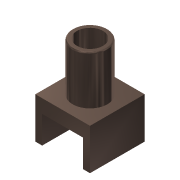
# Autodesk Inventor part: suporte-barra
Saved by Autodesk Inventor 2015 (Build 190159000, 159)
## iProperties
Created: 2016-08-11
Part Number: suporte-barra
Material: Steel, Carbon
Document SubType Name: Modeling
Designer: EriveltonDell
Density: 7.87 g/cm^3
Appearance: Gunmetal - Antique Polished
Mass: 377.778 g
Surface Area: 137.801 cm^2
Volume: 48.0022 cm^3
Author: EriveltonDell
Autodesk Inventor part; units mm, degrees
ref_plane "YZ Plane" through (0, 0, 0) normal (1, 0, 0) x (0, 1, 0)
ref_plane "XZ Plane" through (0, 0, 0) normal (0, 1, 0) x (-1, 0, 0)
ref_plane "XY Plane" through (0, 0, 0) normal (0, 0, 1) x (1, 0, 0)
sketch "Sketch1" plane through (0, 0, 0) normal (0, 1, 0) x (-1, 0, 0)
  line L0 (15, 0) -> (20, 0)
  line L1 (20, 0) -> (20, 20)
  line L2 (20, 20) -> (-20, 20)
  line L3 (-20, 20) -> (-20, 0)
  line L4 (15, 0) -> (15, 10)
  line L5 (15, 10) -> (-15, 10)
  line L6 (-15, 10) -> (-15, 0)
  line L7 (-20, 0) -> (-15, 0)
  line L8 (15, 0) -> (20, 0)
  line L9 (20, 0) -> (20, -10)
  line L10 (20, -10) -> (15, -10)
  line L11 (15, -10) -> (15, 0)
  line L12 (-15, 0) -> (-15, -10)
  line L13 (-15, -10) -> (-20, -10)
  line L14 (-20, -10) -> (-20, 0)
  dimension "d49" = 40
  dimension "d51" = 10
  dimension "d52" = 30
  dimension "d56" = 5
  dimension "d57" = 10
  dimension "d58" = 5
  constraints: 30 end point, 9 perpendicular, 3 collinear, 2 vertical, 1 horizontal, 1 point on line
  measures "d49" distance of L1.end L2.end
  measures "d51" distance of L0.start L4.end
  measures "d52" distance of L4.end L5.end
  measures "d56" distance of L9.end L10.end
  measures "d57" distance of L6.end L12.end
  measures "d58" distance of L12.end L13.end
extrude "Extrusion1" add sketch "Sketch1" along normal mid plane 40
sketch "Sketch6" plane through (0, 0, 0) normal (0, 0, 1) x (1, 0, 0)
  circle A0 centre (0, 0) radius 12.7
  dimension "d33" = 25.4
  constraints: 1 centre point, 1 coincident
  measures "d33" diameter of A0
extrude "Extrusion6" add sketch "Sketch6" along normal blind 55.4
hole "Hole2" at (0, 0, 55.4) direction (0, 0, -1) diameter 19 depth 15
fillet "Fillet3" radius 1 1 edges at (-12.7, 0, 55.4)
sketch "Sketch8" plane through (0, 0, 0) normal (0, 0, -1) x (-1, 0, 0)
  circle A0 centre (0, 0) radius 13
  constraints: 1 centre point, 1 coincident
extrude "Extrusion8" cut sketch "Sketch8" against normal blind 10
body "Solid1"
